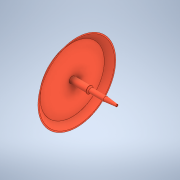
# Autodesk Inventor part: rubber replica
Saved by Autodesk Inventor 2020 (Build 240168000, 168)
## iProperties
Created: 2020-04-08
Part Number: rubber replica
Material: Generic
Document SubType Name: Modeling
Designer: Ben
Density: 1 g/cm^3
Appearance: Default
Author: Ben
Autodesk Inventor part; units mm, degrees
ref_plane "YZ Plane" through (0, 0, 0) normal (1, 0, 0) x (0, 1, 0)
ref_plane "XZ Plane" through (0, 0, 0) normal (0, 1, 0) x (-1, 0, 0)
ref_plane "XY Plane" through (0, 0, 0) normal (0, 0, 1) x (1, 0, 0)
sketch "Sketch1" plane through (0, 0, 0) normal (1, 0, 0) x (0, 1, 0)
  circle A0 centre (0, 0) radius 17
  circle A1 centre (0, 0) radius 14
  dimension "d0" = 34
  dimension "d1" = 28
  constraints: 2 centre point, 2 coincident
  measures "d0" diameter of A0
  measures "d1" diameter of A1
extrude "Extrusion1" add sketch "Sketch1" along normal blind 0.4 contours A1
ref_plane "Work Plane1" through (2.4, 0, 0) normal (1, 0, 0) x (0, 0, -1)
sketch "Sketch2" plane through (2.4, 0, 0) normal (1, 0, 0) x (0, 0, -1)
  circle A0 centre (0, 0) radius 17
  dimension "d5" = 34
  constraints: 1 centre point, 1 coincident
  measures "d5" diameter of A0
sketch "Sketch3" plane through (0, 0, 0) normal (0, 1, 0) x (-1, 0, 0)
  line L0 (-2.4, 17) -> (-2.4, -17) projected
  line L1 (0, 14) -> (0, -14) projected
  line L2 (0, 14) -> (-2.4, 17)
  line L3 (-0.4, 14) -> (-0.4, -14) projected
  line L4 (-0.4, 14) -> (-2.4, 16.5)
  line L5 (-0.4, 0) -> (-1.3096, 0)
  line L6 (0, 14) -> (-0.4, 14)
  line L7 (-2.4, 16.5) -> (-2.4, 17)
  point P0 (0, 0)
  constraints: 10 end point, 2 horizontal, 1 collinear, 1 midpoint, 1 parallel, 1 point on line
revolve "Revolution1" add sketch "Sketch3" angle 360 about axis through (0.4, 0, 0) along (1, 0, 0)
sketch "Sketch4" plane through (0, 0, 0) normal (-1, 0, 0) x (0, 0, 1)
  circle A0 centre (0, 0) radius 14 projected
  circle A1 centre (0, 0) radius 4.5
  dimension "d7" = 9
  constraints: 1 centre point, 1 coincident
  measures "d7" diameter of A1
extrude "Extrusion2" add sketch "Sketch4" along normal blind 0.6 contours A1
fillet "Fillet1" radius 2 1 edges at (0, 0, -4.5)
sketch "Sketch5" plane through (-0.6, 0, 0) normal (-1, 0, 0) x (0, 0, 1)
  circle A0 centre (0, 0) radius 4.5 projected
  circle A1 centre (0, 0) radius 1
  dimension "d11" = 2
  constraints: 1 centre point, 1 coincident
  measures "d11" diameter of A1
extrude "Extrusion3" add sketch "Sketch5" along normal blind 3 contours A1
sketch "Sketch6" plane through (0.4, 0, 0) normal (1, 0, 0) x (0, 0, -1)
  circle A0 centre (0, 0) radius 14 projected
  circle A1 centre (0, 0) radius 1.35
  dimension "d14" = 2.7
  constraints: 1 centre point, 1 coincident
  measures "d14" diameter of A1
extrude "Extrusion4" add sketch "Sketch6" along normal blind 7.5 contours A1
sketch "Sketch7" plane through (7.9, 0, 0) normal (1, 0, 0) x (0, 0, -1)
  circle A0 centre (0, 0) radius 1 projected
  circle A1 centre (0, 0) radius 1.5
  dimension "d17" = 3
  constraints: 1 centre point, 1 coincident
  measures "d17" diameter of A1
extrude "Extrusion5" add sketch "Sketch7" along normal blind 0.14 contours A0 | A1
sketch "Sketch8" plane through (8.04, 0, 0) normal (1, 0, 0) x (0, 0, -1)
  circle A0 centre (0, 0) radius 1.5 projected
  circle A1 centre (0, 0) radius 1
  dimension "d20" = 2
  constraints: 1 centre point, 1 coincident
  measures "d20" diameter of A1
extrude "Extrusion6" add sketch "Sketch8" along normal blind 11.86 contours A1
chamfer "Chamfer1" distance 0.5 angle 45 1 edges at (8.04, 0, 1)
sketch "Sketch9" plane through (0, 0, 0) normal (0, 0, 1) x (1, 0, 0)
  line L0 (19.9, -1) -> (19.9, 1) projected
  line L1 (19.9, -0.5) -> (14.9, -1)
  line L2 (8.54, -1) -> (19.9, -1) projected
  line L3 (19.9, -0.5) -> (19.9, -1)
  line L4 (19.9, -1) -> (15, -1)
  line L5 (23, 0) -> (21.1668, 0)
  point P0 (0, 0)
  dimension "d26" = 0.5
  dimension "d27" = 5
  constraints: 8 end point, 3 point on line, 1 horizontal, 1 vertical
  measures "d26" distance of L0.start L1.start
  measures "d27" distance from line of L0 L1.end
revolve "Revolution2" cut sketch "Sketch9" angle 360 about axis through (23, 0, 0) along (-1, 0, 0)
sketch "Sketch10" plane through (19.9, 0, 0) normal (1, 0, 0) x (0, 0, -1)
  circle A0 centre (0, 0) radius 0.5 projected
  circle A1 centre (0, 0) radius 0.4
  dimension "d29" = 0.8
  constraints: 1 centre point, 1 coincident
  measures "d29" diameter of A1
extrude "Extrusion7" cut sketch "Sketch10" against normal blind 0.1 contours A1
fillet "Fillet2" radius 0.1 1 edges at (19.8, 0, 0.4)
sketch "Sketch11" plane through (-0.6, 0, 0) normal (-1, 0, 0) x (0, 0, 1)
  circle A0 centre (0, 0) radius 1 projected
  circle A1 centre (0, 0) radius 4.5 projected
  circle A2 centre (0, 0) radius 3.25
  dimension "d33" = 6.5
  constraints: 1 centre point, 1 coincident
  measures "d33" diameter of A2
extrude "Extrusion8" add sketch "Sketch11" along normal blind 0.1 contours A2
fillet "Fillet3" radius 0.1 1 edges at (-0.6, 0, -3.25)
body "Solid1"
